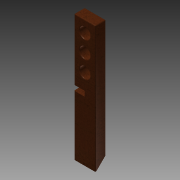
# Autodesk Inventor part: stand1
Saved by Autodesk Inventor 2015 (Build 190159000, 159)
## iProperties
Created: 2014-07-19
Part Number: stand1
Material: Wood (Walnut)
Document SubType Name: Modeling
Designer: pc
Density: 0.55 g/cm^3
Appearance: Walnut - Natural Polished
Author: pc
Autodesk Inventor part; units mm, degrees
ref_plane "YZ Plane" through (0, 0, 0) normal (1, 0, 0) x (0, 1, 0)
ref_plane "XZ Plane" through (0, 0, 0) normal (0, 1, 0) x (-1, 0, 0)
ref_plane "XY Plane" through (0, 0, 0) normal (0, 0, 1) x (1, 0, 0)
sketch "Sketch1" plane through (0, 0, 0) normal (0, 1, 0) x (-1, 0, 0)
  line L0 (25, 150) -> (-25, 150)
  line L1 (-25, 150) -> (-25, -150)
  line L2 (-25, -150) -> (25, -150)
  line L3 (25, -150) -> (25, 150)
  line L4 (25, 150) -> (-25, -150) construction
  line L5 (-25, 150) -> (25, -150) construction
  point P0 (0, 0)
  dimension "d0" = 300
  dimension "d1" = 50
  constraints: 12 end point, 2 midpoint, 2 parallel, 1 horizontal, 1 perpendicular
  measures "d0" distance of L0.end L1.end
  measures "d1" distance of L0.start L0.end
extrude "Extrusion1" add sketch "Sketch1" along normal blind 25
fillet "Fillet4" radius 2 3 edges at (-25, 0, 0) (-25, 12.5, 150) (-25, 25, 0)
sketch "Sketch2" plane through (0, 0, 0) normal (0, -1, 0) x (1, 0, 0)
  circle A0 centre (0, 123) radius 12.5
  circle A1 centre (0, 83) radius 12.5
  circle A2 centre (0, 43) radius 12.5
  line L0 (-23, 148) -> (25, 148) projected
  line L1 (0, 83) -> (0, 43) construction
  line L2 (0, 123) -> (0, 83) construction
  line L3 (0, 0) -> (0, 148) construction
  line L4 (-39.2491, 0) -> (23.3031, 0) construction
  line L5 (0, -6) -> (-25, -6)
  line L6 (-25, -6) -> (-25, 6)
  line L7 (-25, 6) -> (0, 6)
  line L8 (0, 6) -> (0, -6)
  line L9 (0, -6) -> (-25, 6) construction
  line L10 (-25, -6) -> (0, 6) construction
  line L11 (-25, 148) -> (-25, -150) projected
  point P0 (23, 148)
  point P1 (0, 103)
  point P2 (-11.5, 0)
  point P3 (-12.5, 0)
  point P4 (-25, -148)
  dimension "d9" = 25
  dimension "d10" = 25
  dimension "d11" = 25
  dimension "d12" = 40
  dimension "d13" = 40
  dimension "d14" = 25
  dimension "d16" = 12
  constraints: 20 end point, 4 point on line, 3 centre point, 3 midpoint, 2 collinear, 2 horizontal, 2 parallel, 2 vertical, 1 coincident, 1 perpendicular
  measures "d9" diameter of A0
  measures "d10" diameter of A1
  measures "d11" diameter of A2
  measures "d12" distance of L1.start L2.start
  measures "d13" distance of A2.centre L1.start
  measures "d14" distance from line of L2.start L0
  measures "d16" distance between parallel lines of L5 L7
extrude "Extrusion3" cut sketch "Sketch2" against normal through all
fillet "Fillet6" radius 2 1 edges at (-12.5, 0, 43)
fillet "Fillet7" radius 2 1 edges at (-12.5, 0, 83)
fillet "Fillet8" radius 2 1 edges at (-12.5, 0, 123)
fillet "Fillet9" radius 2 1 edges at (-12.5, 25, 123)
fillet "Fillet10" radius 2 1 edges at (-12.5, 25, 83)
fillet "Fillet11" radius 2 1 edges at (-12.5, 25, 43)
sketch "Sketch4" plane through (25, 0, 150) normal (1, 0, 0) x (0, 0, -1)
  line L0 (300, 0) -> (275, 25)
  line L1 (0, 25) -> (300, 25) projected
  line L2 (300, 0) -> (300, 25)
  point P0 (150, 0)
  dimension "d29" = 45
  constraints: 4 end point, 1 perpendicular, 1 point on line
  measures "d29" angle of L1 L0
extrude "Extrusion4" cut sketch "Sketch4" against normal through all
fillet "Fillet12" radius 2 1 edges at (25, 0, 0)
fillet "Fillet13" radius 2 1 edges at (25, 25, 12.5)
fillet "Fillet14" radius 2 8 edges at (25, 12.5, -137.5) (24.4142, 24.4142, -125.5858) (0, 25, -125) (-24.4142, 24.4142, -125.5858) (-25, 12.5, -137.5) (-24.4142, 0.5858, -149.4142) (0, 0, -150) (24.4142, 0.5858, -149.4142)
fillet "Fillet15" radius 2 7 edges at (25, 12.5, 150) (24.4142, 24.4142, 150) (0, 25, 150) (-24.4142, 24.4142, 149.4142) (24.4142, 0.5858, 150) (0, 0, 150) (-24.4142, 0.5858, 149.4142)
equation "\"d13\" = d12"
body "Solid1"
